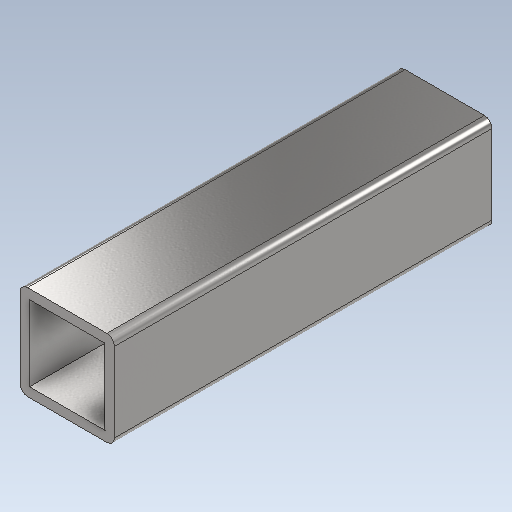
# Autodesk Inventor part: member_axial
Saved by Autodesk Inventor 2021 (Build 250183000, 183)
## iProperties
Created: 2021-06-01
Part Number: member_axial
Material: Steel, Galvanized
Document SubType Name: Modeling
Designer: Watchdog
Density: 7.85 g/cm^3
Appearance: Galvanized
Author: Watchdog
Autodesk Inventor part; units mm, degrees
ref_plane "YZ Plane" through (0, 0, 0) normal (1, 0, 0) x (0, 1, 0)
ref_plane "XZ Plane" through (0, 0, 0) normal (0, 1, 0) x (-1, 0, 0)
ref_plane "XY Plane" through (0, 0, 0) normal (0, 0, 1) x (1, 0, 0)
sketch "Sketch1" plane through (0, 0, 0) normal (0, 0, 1) x (1, 0, 0)
  line L0 (-12.5, 12.5) -> (12.5, 12.5)
  line L1 (12.5, 12.5) -> (12.5, -12.5)
  line L2 (12.5, -12.5) -> (-12.5, -12.5)
  line L3 (-12.5, -12.5) -> (-12.5, 12.5)
  line L4 (10, 10) -> (-10, 10)
  line L5 (-10, 10) -> (-10, -10)
  line L6 (-10, -10) -> (10, -10)
  line L7 (10, -10) -> (10, 10)
  point P0 (0, 0)
  dimension "d0" = 25
  dimension "d1" = 25
  dimension "d2" = 12.5
  dimension "d3" = 12.5
  dimension "d4" = 2.5
  constraints: 16 end point, 4 parallel, 2 perpendicular, 1 horizontal, 3 other
  measures "d0" distance of L0.start L0.end
  measures "d1" distance of L2.end L0.start
  measures "d2" distance from line of point (0, 0) L0
  measures "d3" distance from line of point (0, 0) L3
  measures "d4" distance between parallel lines of L0 L4
extrude "Extrusion1" add sketch "Sketch1" along normal blind 1000
fillet "Fillet1" radius 2 4 edges at (12.5, 12.5, 500) (-12.5, 12.5, 500) (-12.5, -12.5, 500) (12.5, -12.5, 500)
ref_plane "Work Plane1" through (0, 0, 100) normal (0, 0, -1) x (-1, 0, 0)
split "Split1" plane through (0, 0, 100) removes the side toward (0, 0, 1)
ref_plane "axialPlane" through (0, -10.5, 0) normal (1, 0, 0) x (0, 0, -1)
equation "\"d0\" = -2 * a + sm_varx_squareBarDimension - tol"
equation "\"d1\" = d0"
equation "\"d2\" = 0.5 * d1"
equation "\"d3\" = 0.5 * d0"
equation "\"d4\" = sm_varx_squareBarThickness"
equation "\"sm_varx_squareBarThickness\" = 2.5"
equation "\"a\" = sm_varx_squareBarThickness"
equation "\"hoop_angle_z\" = 45deg"
equation "\"hoop_bearing_length\" = 5deg"
equation "\"hoop_cable_diam\" = 5"
equation "\"hoop_cable_pulley_diam\" = 22"
equation "\"hoop_thickness_large\" = 4"
equation "\"hoop_thickness_medium\" = 3.2"
equation "\"hoop_thickness_small\" = 2"
equation "\"hoop_width_large\" = 51"
equation "\"hoop_width_medium\" = 33.7"
equation "\"hoop_width_small\" = 25.4"
equation "\"rack_tooth_addendum\" = 5"
equation "\"rack_tooth_dedendum\" = 5"
equation "\"rack_tooth_thickness\" = 5"
equation "\"secure_arm_angle\" = 35deg"
equation "\"secure_arm_radii\" = 9"
equation "\"support_baseClamp_platformLengthBuffer\" = 35"
equation "\"support_baseClamp_platformThickness\" = 15"
equation "\"support_baseClamp_platformWidthBuffer\" = 0"
equation "\"support_baseClamp_sleeveHoleDiameter\" = 12"
equation "\"support_baseClamp_sleeveSweepTerminationAngle\" = 55deg"
equation "\"support_baseClamp_thickness\" = 8"
equation "\"support_frame_endHoleBuffer\" = 45"
equation "\"support_frame_squareBarFillet\" = 2"
equation "\"support_frame_squareBarThickness\" = 5"
equation "\"hoop_tabs_thickness\" = 6"
equation "\"hoop_tabs_hole\" = 12"
equation "\"wheelchair_deployed_width\" = 635"
equation "\"wheelchair_deployed_length\" = 1067"
equation "\"wheelchair_deployed_height\" = 914"
equation "\"sm_varx_pinPlate_thickness\" = 5"
equation "\"sm_varx_pinPlate_holeDiameter\" = 5"
equation "\"sm_varx_member_tolerance\" = 0"
equation "\"hoop_bushing12_radialInterference\" = 0"
equation "\"hoop_bushing23_radialInterference\" = 0"
equation "\"hoop_bushing23_od\" = -2 * hoop_thickness_medium + hoop_width_medium + hoop_bushing23_radialInterference"
equation "\"hoop_bushing23_thickness\" = -hoop_width_small + hoop_bushing23_od - 2 * hoop_bushing23_radialInterference"
equation "\"hoop_bushing12_od\" = -2 * hoop_thickness_large + hoop_width_large + hoop_bushing12_radialInterference"
equation "\"wheelchatir_pos_deploy_angle_0\" = 65deg"
equation "\"wheelchatir_pos_store_angle_0\" = 90deg"
equation "\"wheelchatir_pos_deploy_angle_1\" = 20deg"
equation "\"wheelchatir_pos_store_angle_1\" = 20deg"
equation "\"hoop_bushing12_thickness\" = -hoop_width_medium + hoop_bushing12_od - 2 * hoop_bushing12_radialInterference"
equation "\"sm_varx_squareBarDimension\" = 30"
equation "\"tol\" = 0"
body "Solid1"
